Autodesk Fusion 360 part; units mm, degrees
(part 3 of 7)
  line L359 (74.972, -60.812) -> (75.0961, -60.7061)
  line L360 (75.0961, -60.7061) -> (75.2145, -60.5939)
  line L361 (75.2145, -60.5939) -> (75.3268, -60.4755)
  line L362 (75.3268, -60.4755) -> (75.4327, -60.3513)
  line L363 (75.4327, -60.3513) -> (75.6604, -60.5355)
  line L364 (75.6604, -60.5355) -> (75.7298, -60.5765)
  line L365 (75.7298, -60.5765) -> (75.8054, -60.6096)
  line L366 (75.8054, -60.6096) -> (75.8853, -60.6371)
  line L367 (75.8853, -60.6371) -> (75.9686, -60.6597)
  line L368 (75.9686, -60.6597) -> (76.0549, -60.6779)
  line L369 (76.0549, -60.6779) -> (76.1439, -60.6917)
  line L370 (76.1439, -60.6917) -> (76.2354, -60.7014)
  line L371 (76.2354, -60.7014) -> (76.3291, -60.707)
  line L372 (76.3291, -60.707) -> (76.4248, -60.7085)
  line L373 (76.4248, -60.7085) -> (76.5224, -60.7059)
  line L374 (76.5224, -60.7059) -> (76.6217, -60.6994)
  line L375 (76.6217, -60.6994) -> (76.7225, -60.6887)
  line L376 (76.7225, -60.6887) -> (76.7666, -60.6157)
  line L377 (76.7666, -60.6157) -> (76.8092, -60.5419)
  line L378 (76.8092, -60.5419) -> (76.8504, -60.4672)
  line L379 (76.8504, -60.4672) -> (76.8092, -60.3745)
  line L380 (76.8092, -60.3745) -> (76.7652, -60.2853)
  line L381 (76.7652, -60.2853) -> (76.7187, -60.1995)
  line L382 (76.7187, -60.1995) -> (76.6695, -60.1173)
  line L383 (76.6695, -60.1173) -> (76.6178, -60.039)
  line L384 (76.6178, -60.039) -> (76.5637, -59.9646)
  line L385 (76.5637, -59.9646) -> (76.5072, -59.8945)
  line L386 (76.5072, -59.8945) -> (76.4483, -59.8288)
  line L387 (76.4483, -59.8288) -> (76.3871, -59.7679)
  line L388 (76.3871, -59.7679) -> (76.3233, -59.7126)
  line L389 (76.3233, -59.7126) -> (76.2568, -59.6636)
  line L390 (76.2568, -59.6636) -> (76.1866, -59.6241)
  line L391 (76.1866, -59.6241) -> (75.9133, -59.5189)
  line L392 (75.9133, -59.5189) -> (75.9679, -59.3651)
  line L393 (75.9679, -59.3651) -> (76.0142, -59.2086)
  line L394 (76.0142, -59.2086) -> (76.0523, -59.05)
  line L395 (76.0523, -59.05) -> (76.0819, -58.8895)
  circle A0 centre (73.0295, -58.4089) radius 2.2
extrude "Extrude2" add sketch "Sketch2" along normal blind 2 separate body makes body 3 in component "CT idler 1"
combine "Combine1" operation add target body 2 tool bodies 3 makes body 4 at (74.9068, -57.2617, 40.3333) in component "CT idler 1"
ref_plane "WorkPlane1" through (0, 0, 39) normal (0, 0, 1) x (1, 0, 0) in component "CT idler 2"
sketch "Sketch1 (3)" plane through (0, 0, 39) normal (0, 0, 1) x (1, 0, 0) in component "CT idler 2"
  line L0 (68.9168, -62.2983) -> (69.3634, -62.3215)
  line L1 (69.3634, -62.3215) -> (69.4355, -62.319)
  line L2 (69.4355, -62.319) -> (69.5079, -62.3112)
  line L3 (69.5079, -62.3112) -> (69.5805, -62.2999)
  line L4 (69.5805, -62.2999) -> (69.6531, -62.2856)
  line L5 (69.6531, -62.2856) -> (69.7259, -62.2688)
  line L6 (69.7259, -62.2688) -> (69.7986, -62.2497)
  line L7 (69.7986, -62.2497) -> (69.8714, -62.2283)
  line L8 (69.8714, -62.2283) -> (69.9443, -62.205)
  line L9 (69.9443, -62.205) -> (70.0171, -62.1796)
  line L10 (70.0171, -62.1796) -> (70.0898, -62.1524)
  line L11 (70.0898, -62.1524) -> (70.1626, -62.1234)
  line L12 (70.1626, -62.1234) -> (70.2352, -62.0926)
  line L13 (70.2352, -62.0926) -> (70.2374, -61.9521)
  line L14 (70.2374, -61.9521) -> (70.2374, -61.8117)
  line L15 (70.2374, -61.8117) -> (70.2352, -61.6713)
  line L16 (70.2352, -61.6713) -> (70.1626, -61.6405)
  line L17 (70.1626, -61.6405) -> (70.0898, -61.6115)
  line L18 (70.0898, -61.6115) -> (70.0171, -61.5842)
  line L19 (70.0171, -61.5842) -> (69.9443, -61.5589)
  line L20 (69.9443, -61.5589) -> (69.8714, -61.5355)
  line L21 (69.8714, -61.5355) -> (69.7986, -61.5142)
  line L22 (69.7986, -61.5142) -> (69.7259, -61.4951)
  line L23 (69.7259, -61.4951) -> (69.6531, -61.4782)
  line L24 (69.6531, -61.4782) -> (69.5805, -61.464)
  line L25 (69.5805, -61.464) -> (69.5079, -61.4527)
  line L26 (69.5079, -61.4527) -> (69.4355, -61.4449)
  line L27 (69.4355, -61.4449) -> (69.3634, -61.4423)
  line L28 (69.3634, -61.4423) -> (68.9168, -61.4656)
  line L29 (68.9168, -61.4656) -> (68.903, -61.2549)
  line L30 (68.903, -61.2549) -> (68.8837, -61.0447)
  line L31 (68.8837, -61.0447) -> (68.8589, -60.835)
  line L32 (68.8589, -60.835) -> (68.8286, -60.6261)
  line L33 (68.8286, -60.6261) -> (69.2703, -60.5559)
  line L34 (69.2703, -60.5559) -> (69.3403, -60.5385)
  line L35 (69.3403, -60.5385) -> (69.4095, -60.5158)
  line L36 (69.4095, -60.5158) -> (69.4781, -60.4896)
  line L37 (69.4781, -60.4896) -> (69.5462, -60.4606)
  line L38 (69.5462, -60.4606) -> (69.6138, -60.429)
  line L39 (69.6138, -60.429) -> (69.681, -60.3952)
  line L40 (69.681, -60.3952) -> (69.7478, -60.3592)
  line L41 (69.7478, -60.3592) -> (69.8142, -60.3211)
  line L42 (69.8142, -60.3211) -> (69.8801, -60.2812)
  line L43 (69.8801, -60.2812) -> (69.9456, -60.2395)
  line L44 (69.9456, -60.2395) -> (70.0107, -60.1959)
  line L45 (70.0107, -60.1959) -> (70.0754, -60.1507)
  line L46 (70.0754, -60.1507) -> (70.0483, -60.0129)
  line L47 (70.0483, -60.0129) -> (70.0191, -59.8756)
  line L48 (70.0191, -59.8756) -> (69.9878, -59.7387)
  line L49 (69.9878, -59.7387) -> (69.9104, -59.7236)
  line L50 (69.9104, -59.7236) -> (69.8332, -59.7104)
  line L51 (69.8332, -59.7104) -> (69.7563, -59.6989)
  line L52 (69.7563, -59.6989) -> (69.6798, -59.6892)
  line L53 (69.6798, -59.6892) -> (69.6038, -59.6815)
  line L54 (69.6038, -59.6815) -> (69.5281, -59.6758)
  line L55 (69.5281, -59.6758) -> (69.4529, -59.6722)
  line L56 (69.4529, -59.6722) -> (69.3783, -59.6709)
  line L57 (69.3783, -59.6709) -> (69.3043, -59.672)
  line L58 (69.3043, -59.672) -> (69.231, -59.676)
  line L59 (69.231, -59.676) -> (69.1585, -59.6834)
  line L60 (69.1585, -59.6834) -> (69.0875, -59.696)
  line L61 (69.0875, -59.696) -> (68.6554, -59.8116)
  line L62 (68.6554, -59.8116) -> (68.5982, -59.6083)
  line L63 (68.5982, -59.6083) -> (68.5356, -59.4067)
  line L64 (68.5356, -59.4067) -> (68.4677, -59.2068)
  line L65 (68.4677, -59.2068) -> (68.3946, -59.0087)
  line L66 (68.3946, -59.0087) -> (68.812, -58.8483)
  line L67 (68.812, -58.8483) -> (68.8769, -58.8167)
  line L68 (68.8769, -58.8167) -> (68.9399, -58.7801)
  line L69 (68.9399, -58.7801) -> (69.0015, -58.7402)
  line L70 (69.0015, -58.7402) -> (69.0621, -58.6977)
  line L71 (69.0621, -58.6977) -> (69.1217, -58.6527)
  line L72 (69.1217, -58.6527) -> (69.1804, -58.6056)
  line L73 (69.1804, -58.6056) -> (69.2382, -58.5565)
  line L74 (69.2382, -58.5565) -> (69.2952, -58.5056)
  line L75 (69.2952, -58.5056) -> (69.3515, -58.4528)
  line L76 (69.3515, -58.4528) -> (69.4069, -58.3983)
  line L77 (69.4069, -58.3983) -> (69.4615, -58.3422)
  line L78 (69.4615, -58.3422) -> (69.5154, -58.2845)
  line L79 (69.5154, -58.2845) -> (69.4602, -58.1554)
  line L80 (69.4602, -58.1554) -> (69.4031, -58.0271)
  line L81 (69.4031, -58.0271) -> (69.344, -57.8997)
  line L82 (69.344, -57.8997) -> (69.2651, -57.9011)
  line L83 (69.2651, -57.9011) -> (69.1869, -57.9042)
  line L84 (69.1869, -57.9042) -> (69.1093, -57.9089)
  line L85 (69.1093, -57.9089) -> (69.0325, -57.9154)
  line L86 (69.0325, -57.9154) -> (68.9564, -57.9236)
  line L87 (68.9564, -57.9236) -> (68.8813, -57.9338)
  line L88 (68.8813, -57.9338) -> (68.807, -57.9459)
  line L89 (68.807, -57.9459) -> (68.7337, -57.9601)
  line L90 (68.7337, -57.9601) -> (68.6615, -57.9766)
  line L91 (68.6615, -57.9766) -> (68.5907, -57.9958)
  line L92 (68.5907, -57.9958) -> (68.5214, -58.0181)
  line L93 (68.5214, -58.0181) -> (68.4544, -58.0451)
  line L94 (68.4544, -58.0451) -> (68.0559, -58.248)
  line L95 (68.0559, -58.248) -> (67.9576, -58.0611)
  line L96 (67.9576, -58.0611) -> (67.8545, -57.8769)
  line L97 (67.8545, -57.8769) -> (67.7465, -57.6955)
  line L98 (67.7465, -57.6955) -> (67.6338, -57.517)
  line L99 (67.6338, -57.517) -> (68.0088, -57.2733)
  line L100 (68.0088, -57.2733) -> (68.0657, -57.2288)
  line L101 (68.0657, -57.2288) -> (68.1196, -57.1799)
  line L102 (68.1196, -57.1799) -> (68.1717, -57.1281)
  line L103 (68.1717, -57.1281) -> (68.2221, -57.0739)
  line L104 (68.2221, -57.0739) -> (68.271, -57.0176)
  line L105 (68.271, -57.0176) -> (68.3187, -56.9593)
  line L106 (68.3187, -56.9593) -> (68.365, -56.8993)
  line L107 (68.365, -56.8993) -> (68.4102, -56.8375)
  line L108 (68.4102, -56.8375) -> (68.4542, -56.7742)
  line L109 (68.4542, -56.7742) -> (68.4971, -56.7094)
  line L110 (68.4971, -56.7094) -> (68.5389, -56.6432)
  line L111 (68.5389, -56.6432) -> (68.5795, -56.5756)
  line L112 (68.5795, -56.5756) -> (68.4987, -56.4607)
  line L113 (68.4987, -56.4607) -> (68.4162, -56.3471)
  line L114 (68.4162, -56.3471) -> (68.3319, -56.2348)
  line L115 (68.3319, -56.2348) -> (68.255, -56.2526)
  line L116 (68.255, -56.2526) -> (68.1791, -56.2718)
  line L117 (68.1791, -56.2718) -> (68.1043, -56.2926)
  line L118 (68.1043, -56.2926) -> (68.0305, -56.3149)
  line L119 (68.0305, -56.3149) -> (67.9578, -56.3388)
  line L120 (67.9578, -56.3388) -> (67.8864, -56.3643)
  line L121 (67.8864, -56.3643) -> (67.8162, -56.3916)
  line L122 (67.8162, -56.3916) -> (67.7475, -56.4207)
  line L123 (67.7475, -56.4207) -> (67.6804, -56.4519)
  line L124 (67.6804, -56.4519) -> (67.615, -56.4854)
  line L125 (67.615, -56.4854) -> (67.5519, -56.5216)
  line L126 (67.5519, -56.5216) -> (67.492, -56.562)
  line L127 (67.492, -56.562) -> (67.1444, -56.8433)
  line L128 (67.1444, -56.8433) -> (67.0094, -56.6809)
  line L129 (67.0094, -56.6809) -> (66.8702, -56.5222)
  line L130 (66.8702, -56.5222) -> (66.7269, -56.3672)
  line L131 (66.7269, -56.3672) -> (66.5795, -56.216)
  line L132 (66.5795, -56.216) -> (66.8957, -55.8996)
  line L133 (66.8957, -55.8996) -> (66.942, -55.8443)
  line L134 (66.942, -55.8443) -> (66.9847, -55.7853)
  line L135 (66.9847, -55.7853) -> (67.0248, -55.7238)
  line L136 (67.0248, -55.7238) -> (67.0628, -55.6603)
  line L137 (67.0628, -55.6603) -> (67.099, -55.595)
  line L138 (67.099, -55.595) -> (67.1335, -55.5281)
  line L139 (67.1335, -55.5281) -> (67.1663, -55.4597)
  line L140 (67.1663, -55.4597) -> (67.1977, -55.39)
  line L141 (67.1977, -55.39) -> (67.2276, -55.3189)
  line L142 (67.2276, -55.3189) -> (67.256, -55.2466)
  line L143 (67.256, -55.2466) -> (67.2831, -55.1731)
  line L144 (67.2831, -55.1731) -> (67.3089, -55.0985)
  line L145 (67.3089, -55.0985) -> (67.2059, -55.003)
  line L146 (67.2059, -55.003) -> (67.1016, -54.909)
  line L147 (67.1016, -54.909) -> (66.9958, -54.8166)
  line L148 (66.9958, -54.8166) -> (66.9243, -54.85)
  line L149 (66.9243, -54.85) -> (66.854, -54.8847)
  line L150 (66.854, -54.8847) -> (66.7851, -54.9205)
  line L151 (66.7851, -54.9205) -> (66.7176, -54.9577)
  line L152 (66.7176, -54.9577) -> (66.6515, -54.9962)
  line L153 (66.6515, -54.9962) -> (66.5869, -55.036)
  line L154 (66.5869, -55.036) -> (66.524, -55.0773)
  line L155 (66.524, -55.0773) -> (66.4628, -55.1201)
  line L156 (66.4628, -55.1201) -> (66.4036, -55.1645)
  line L157 (66.4036, -55.1645) -> (66.3467, -55.2109)
  line L158 (66.3467, -55.2109) -> (66.2924, -55.2594)
  line L159 (66.2924, -55.2594) -> (66.2423, -55.3113)
  line L160 (66.2423, -55.3113) -> (65.9607, -55.6588)
  line L161 (65.9607, -55.6588) -> (65.7949, -55.528)
  line L162 (65.7949, -55.528) -> (65.6258, -55.4017)
  line L163 (65.6258, -55.4017) -> (65.4534, -55.2799)
  line L164 (65.4534, -55.2799) -> (65.2778, -55.1626)
  line L165 (65.2778, -55.1626) -> (65.5212, -54.7875)
  line L166 (65.5212, -54.7875) -> (65.5551, -54.7237)
  line L167 (65.5551, -54.7237) -> (65.5845, -54.6571)
  line L168 (65.5845, -54.6571) -> (65.611, -54.5886)
  line L169 (65.611, -54.5886) -> (65.635, -54.5186)
  line L170 (65.635, -54.5186) -> (65.6568, -54.4472)
  line L171 (65.6568, -54.4472) -> (65.6766, -54.3746)
  line L172 (65.6766, -54.3746) -> (65.6945, -54.3009)
  line L173 (65.6945, -54.3009) -> (65.7107, -54.2261)
  line L174 (65.7107, -54.2261) -> (65.7251, -54.1504)
  line L175 (65.7251, -54.1504) -> (65.738, -54.0738)
  line L176 (65.738, -54.0738) -> (65.7492, -53.9963)
  line L177 (65.7492, -53.9963) -> (65.7588, -53.9179)
  line L178 (65.7588, -53.9179) -> (65.6383, -53.8459)
  line L179 (65.6383, -53.8459) -> (65.5167, -53.7757)
  line L180 (65.5167, -53.7757) -> (65.394, -53.7073)
  line L181 (65.394, -53.7073) -> (65.331, -53.7549)
  line L182 (65.331, -53.7549) -> (65.2695, -53.8033)
  line L183 (65.2695, -53.8033) -> (65.2095, -53.8527)
  line L184 (65.2095, -53.8527) -> (65.1512, -53.9031)
  line L185 (65.1512, -53.9031) -> (65.0945, -53.9545)
  line L186 (65.0945, -53.9545) -> (65.0397, -54.0069)
  line L187 (65.0397, -54.0069) -> (64.9867, -54.0603)
  line L188 (64.9867, -54.0603) -> (64.9358, -54.1149)
  line L189 (64.9358, -54.1149) -> (64.8871, -54.1707)
  line L190 (64.8871, -54.1707) -> (64.841, -54.2279)
  line L191 (64.841, -54.2279) -> (64.7981, -54.2867)
  line L192 (64.7981, -54.2867) -> (64.7598, -54.3479)
  line L193 (64.7598, -54.3479) -> (64.5566, -54.7463)
  line L194 (64.5566, -54.7463) -> (64.3673, -54.6528)
  line L195 (64.3673, -54.6528) -> (64.1756, -54.5644)
  line L196 (64.1756, -54.5644) -> (63.9816, -54.4811)
  line L197 (63.9816, -54.4811) -> (63.7855, -54.4029)
  line L198 (63.7855, -54.4029) -> (63.9456, -53.9853)
  line L199 (63.9456, -53.9853) -> (63.9655, -53.916)
  line L200 (63.9655, -53.916) -> (63.9804, -53.8447)
  line L201 (63.9804, -53.8447) -> (63.9921, -53.7722)
  line L202 (63.9921, -53.7722) -> (64.001, -53.6987)
  line L203 (64.001, -53.6987) -> (64.0075, -53.6244)
  line L204 (64.0075, -53.6244) -> (64.0117, -53.5492)
  line L205 (64.0117, -53.5492) -> (64.014, -53.4734)
  line L206 (64.014, -53.4734) -> (64.0142, -53.3969)
  line L207 (64.0142, -53.3969) -> (64.0126, -53.3198)
  line L208 (64.0126, -53.3198) -> (64.0092, -53.2422)
  line L209 (64.0092, -53.2422) -> (64.0041, -53.1641)
  line L210 (64.0041, -53.1641) -> (63.9972, -53.0854)
  line L211 (63.9972, -53.0854) -> (63.8644, -53.04)
  line L212 (63.8644, -53.04) -> (63.7308, -52.9966)
  line L213 (63.7308, -52.9966) -> (63.5966, -52.9553)
  line L214 (63.5966, -52.9553) -> (63.5449, -53.0149)
  line L215 (63.5449, -53.0149) -> (63.4948, -53.0751)
  line L216 (63.4948, -53.0751) -> (63.4464, -53.1359)
  line L217 (63.4464, -53.1359) -> (63.3998, -53.1973)
  line L218 (63.3998, -53.1973) -> (63.3551, -53.2593)
  line L219 (63.3551, -53.2593) -> (63.3123, -53.322)
  line L220 (63.3123, -53.322) -> (63.2716, -53.3853)
  line L221 (63.2716, -53.3853) -> (63.2331, -53.4492)
  line L222 (63.2331, -53.4492) -> (63.1971, -53.5139)
  line L223 (63.1971, -53.5139) -> (63.1639, -53.5794)
  line L224 (63.1639, -53.5794) -> (63.1341, -53.6458)
  line L225 (63.1341, -53.6458) -> (63.1094, -53.7137)
  line L226 (63.1094, -53.7137) -> (62.9935, -54.1456)
  line L227 (62.9935, -54.1456) -> (62.7889, -54.0936)
  line L228 (62.7889, -54.0936) -> (62.583, -54.047)
  line L229 (62.583, -54.047) -> (62.3759, -54.0058)
  line L230 (62.3759, -54.0058) -> (62.1678, -53.9701)
  line L231 (62.1678, -53.9701) -> (62.2376, -53.5283)
  line L232 (62.2376, -53.5283) -> (62.2427, -53.4564)
  line L233 (62.2427, -53.4564) -> (62.2425, -53.3835)
  line L234 (62.2425, -53.3835) -> (62.2388, -53.3102)
  line L235 (62.2388, -53.3102) -> (62.2322, -53.2365)
  line L236 (62.2322, -53.2365) -> (62.2231, -53.1624)
  line L237 (62.2231, -53.1624) -> (62.2117, -53.088)
  line L238 (62.2117, -53.088) -> (62.1981, -53.0134)
  line L239 (62.1981, -53.0134) -> (62.1824, -52.9385)
  line L240 (62.1824, -52.9385) -> (62.1648, -52.8635)
  line L241 (62.1648, -52.8635) -> (62.1454, -52.7882)
  line L242 (62.1454, -52.7882) -> (62.1241, -52.7129)
  line L243 (62.1241, -52.7129) -> (62.1011, -52.6374)
  line L244 (62.1011, -52.6374) -> (61.9616, -52.6206)
  line L245 (61.9616, -52.6206) -> (61.822, -52.6059)
  line L246 (61.822, -52.6059) -> (61.6821, -52.5933)
  line L247 (61.6821, -52.5933) -> (61.6439, -52.6624)
  line L248 (61.6439, -52.6624) -> (61.6074, -52.7317)
  line L249 (61.6074, -52.7317) -> (61.5727, -52.8012)
  line L250 (61.5727, -52.8012) -> (61.5399, -52.871)
  line L251 (61.5399, -52.871) -> (61.509, -52.941)
  line L252 (61.509, -52.941) -> (61.4802, -53.0111)
  line L253 (61.4802, -53.0111) -> (61.4536, -53.0815)
  line L254 (61.4536, -53.0815) -> (61.4293, -53.1521)
  line L255 (61.4293, -53.1521) -> (61.4075, -53.2229)
  line L256 (61.4075, -53.2229) -> (61.3886, -53.2938)
  line L257 (61.3886, -53.2938) -> (61.3733, -53.365)
  line L258 (61.3733, -53.365) -> (61.3633, -53.4364)
  line L259 (61.3633, -53.4364) -> (61.3397, -53.8831)
  line L260 (61.3397, -53.8831) -> (61.1287, -53.8747)
  line L261 (61.1287, -53.8747) -> (60.9176, -53.8719)
  line L262 (60.9176, -53.8719) -> (60.7065, -53.8747)
  line L263 (60.7065, -53.8747) -> (60.4956, -53.8831)
  line L264 (60.4956, -53.8831) -> (60.472, -53.4364)
  line L265 (60.472, -53.4364) -> (60.4619, -53.365)
  line L266 (60.4619, -53.365) -> (60.4466, -53.2938)
  line L267 (60.4466, -53.2938) -> (60.4277, -53.2229)
  line L268 (60.4277, -53.2229) -> (60.406, -53.1521)
  line L269 (60.406, -53.1521) -> (60.3817, -53.0815)
  line L270 (60.3817, -53.0815) -> (60.355, -53.0111)
  line L271 (60.355, -53.0111) -> (60.3262, -52.941)
  line L272 (60.3262, -52.941) -> (60.2953, -52.871)
  line L273 (60.2953, -52.871) -> (60.2625, -52.8012)
  line L274 (60.2625, -52.8012) -> (60.2278, -52.7317)
  line L275 (60.2278, -52.7317) -> (60.1914, -52.6624)
  line L276 (60.1914, -52.6624) -> (60.1531, -52.5933)
  line L277 (60.1531, -52.5933) -> (60.0133, -52.6059)
  line L278 (60.0133, -52.6059) -> (59.8736, -52.6206)
  line L279 (59.8736, -52.6206) -> (59.7342, -52.6374)
  line L280 (59.7342, -52.6374) -> (59.7112, -52.7129)
  line L281 (59.7112, -52.7129) -> (59.6899, -52.7882)
  line L282 (59.6899, -52.7882) -> (59.6704, -52.8635)
  line L283 (59.6704, -52.8635) -> (59.6528, -52.9385)
  line L284 (59.6528, -52.9385) -> (59.6372, -53.0134)
  line L285 (59.6372, -53.0134) -> (59.6236, -53.088)
  line L286 (59.6236, -53.088) -> (59.6122, -53.1624)
  line L287 (59.6122, -53.1624) -> (59.603, -53.2365)
  line L288 (59.603, -53.2365) -> (59.5965, -53.3102)
  line L289 (59.5965, -53.3102) -> (59.5928, -53.3835)
  line L290 (59.5928, -53.3835) -> (59.5926, -53.4564)
  line L291 (59.5926, -53.4564) -> (59.5976, -53.5283)
  line L292 (59.5976, -53.5283) -> (59.6674, -53.9701)
  line L293 (59.6674, -53.9701) -> (59.4593, -54.0058)
  line L294 (59.4593, -54.0058) -> (59.2523, -54.047)
  line L295 (59.2523, -54.047) -> (59.0463, -54.0936)
  line L296 (59.0463, -54.0936) -> (58.8417, -54.1456)
  line L297 (58.8417, -54.1456) -> (58.7258, -53.7137)
  line L298 (58.7258, -53.7137) -> (58.7011, -53.6458)
  line L299 (58.7011, -53.6458) -> (58.6713, -53.5794)
  line L300 (58.6713, -53.5794) -> (58.6381, -53.5139)
  line L301 (58.6381, -53.5139) -> (58.6021, -53.4492)
  line L302 (58.6021, -53.4492) -> (58.5637, -53.3853)
  line L303 (58.5637, -53.3853) -> (58.523, -53.322)
  line L304 (58.523, -53.322) -> (58.4802, -53.2593)
  line L305 (58.4802, -53.2593) -> (58.4355, -53.1973)
  line L306 (58.4355, -53.1973) -> (58.3889, -53.1359)
  line L307 (58.3889, -53.1359) -> (58.3405, -53.0751)
  line L308 (58.3405, -53.0751) -> (58.2904, -53.0149)
  line L309 (58.2904, -53.0149) -> (58.2386, -52.9553)
  line L310 (58.2386, -52.9553) -> (58.1044, -52.9966)
  line L311 (58.1044, -52.9966) -> (57.9709, -53.04)
  line L312 (57.9709, -53.04) -> (57.838, -53.0854)
  line L313 (57.838, -53.0854) -> (57.8312, -53.1641)
  line L314 (57.8312, -53.1641) -> (57.826, -53.2422)
  line L315 (57.826, -53.2422) -> (57.8226, -53.3198)
  line L316 (57.8226, -53.3198) -> (57.821, -53.3969)
  line L317 (57.821, -53.3969) -> (57.8213, -53.4734)
  line L318 (57.8213, -53.4734) -> (57.8235, -53.5492)
  line L319 (57.8235, -53.5492) -> (57.8278, -53.6244)
  line L320 (57.8278, -53.6244) -> (57.8343, -53.6987)
  line L321 (57.8343, -53.6987) -> (57.8432, -53.7722)
  line L322 (57.8432, -53.7722) -> (57.8548, -53.8447)
  line L323 (57.8548, -53.8447) -> (57.8698, -53.916)
  line L324 (57.8698, -53.916) -> (57.8896, -53.9853)
  line L325 (57.8896, -53.9853) -> (58.0498, -54.4029)
  line L326 (58.0498, -54.4029) -> (57.8537, -54.4811)
  line L327 (57.8537, -54.4811) -> (57.6597, -54.5644)
  line L328 (57.6597, -54.5644) -> (57.4679, -54.6528)
  line L329 (57.4679, -54.6528) -> (57.2786, -54.7463)
  line L330 (57.2786, -54.7463) -> (57.0754, -54.3479)
  line L331 (57.0754, -54.3479) -> (57.0372, -54.2867)
  line L332 (57.0372, -54.2867) -> (56.9942, -54.2279)
  line L333 (56.9942, -54.2279) -> (56.9481, -54.1707)
  line L334 (56.9481, -54.1707) -> (56.8995, -54.1149)
  line L335 (56.8995, -54.1149) -> (56.8486, -54.0603)
  line L336 (56.8486, -54.0603) -> (56.7956, -54.0069)
  line L337 (56.7956, -54.0069) -> (56.7407, -53.9545)
  line L338 (56.7407, -53.9545) -> (56.6841, -53.9031)
  line L339 (56.6841, -53.9031) -> (56.6257, -53.8527)
  line L340 (56.6257, -53.8527) -> (56.5657, -53.8033)
  line L341 (56.5657, -53.8033) -> (56.5042, -53.7549)
  line L342 (56.5042, -53.7549) -> (56.4412, -53.7073)
  line L343 (56.4412, -53.7073) -> (56.3186, -53.7757)
  line L344 (56.3186, -53.7757) -> (56.1969, -53.8459)
  line L345 (56.1969, -53.8459) -> (56.0764, -53.9179)
  line L346 (56.0764, -53.9179) -> (56.0861, -53.9963)
  line L347 (56.0861, -53.9963) -> (56.0973, -54.0738)
  line L348 (56.0973, -54.0738) -> (56.1101, -54.1504)
  line L349 (56.1101, -54.1504) -> (56.1246, -54.2261)
  line L350 (56.1246, -54.2261) -> (56.1407, -54.3009)
  line L351 (56.1407, -54.3009) -> (56.1587, -54.3746)
  line L352 (56.1587, -54.3746) -> (56.1785, -54.4472)
  line L353 (56.1785, -54.4472) -> (56.2003, -54.5186)
  line L354 (56.2003, -54.5186) -> (56.2243, -54.5886)
  line L355 (56.2243, -54.5886) -> (56.2507, -54.6571)
  line L356 (56.2507, -54.6571) -> (56.2801, -54.7237)
  line L357 (56.2801, -54.7237) -> (56.314, -54.7875)
  line L358 (56.314, -54.7875) -> (56.5575, -55.1626)
  line L359 (56.5575, -55.1626) -> (56.3819, -55.2799)
  line L360 (56.3819, -55.2799) -> (56.2095, -55.4017)
  line L361 (56.2095, -55.4017) -> (56.0403, -55.528)
  line L362 (56.0403, -55.528) -> (55.8745, -55.6588)
  line L363 (55.8745, -55.6588) -> (55.593, -55.3113)
  line L364 (55.593, -55.3113) -> (55.5428, -55.2594)
  line L365 (55.5428, -55.2594) -> (55.4886, -55.2109)
  line L366 (55.4886, -55.2109) -> (55.4316, -55.1645)
  line L367 (55.4316, -55.1645) -> (55.3724, -55.1201)
  line L368 (55.3724, -55.1201) -> (55.3113, -55.0773)
  line L369 (55.3113, -55.0773) -> (55.2483, -55.036)
  line L370 (55.2483, -55.036) -> (55.1838, -54.9962)
  line L371 (55.1838, -54.9962) -> (55.1177, -54.9577)
  line L372 (55.1177, -54.9577) -> (55.0501, -54.9205)
  line L373 (55.0501, -54.9205) -> (54.9812, -54.8847)
  line L374 (54.9812, -54.8847) -> (54.911, -54.85)
  line L375 (54.911, -54.85) -> (54.8394, -54.8166)
  line L376 (54.8394, -54.8166) -> (54.7337, -54.909)
  line L377 (54.7337, -54.909) -> (54.6293, -55.003)
  line L378 (54.6293, -55.003) -> (54.5264, -55.0985)
  line L379 (54.5264, -55.0985) -> (54.5521, -55.1731)
  line L380 (54.5521, -55.1731) -> (54.5792, -55.2466)
  line L381 (54.5792, -55.2466) -> (54.6077, -55.3189)
  line L382 (54.6077, -55.3189) -> (54.6376, -55.39)
  line L383 (54.6376, -55.39) -> (54.6689, -55.4597)
  line L384 (54.6689, -55.4597) -> (54.7018, -55.5281)
  line L385 (54.7018, -55.5281) -> (54.7363, -55.595)
  line L386 (54.7363, -55.595) -> (54.7724, -55.6603)
  line L387 (54.7724, -55.6603) -> (54.8105, -55.7238)
  line L388 (54.8105, -55.7238) -> (54.8506, -55.7853)
  line L389 (54.8506, -55.7853) -> (54.8932, -55.8443)
  line L390 (54.8932, -55.8443) -> (54.9396, -55.8996)
  line L391 (54.9396, -55.8996) -> (55.2557, -56.216)
  line L392 (55.2557, -56.216) -> (55.1084, -56.3672)
  line L393 (55.1084, -56.3672) -> (54.965, -56.5222)
  line L394 (54.965, -56.5222) -> (54.8258, -56.6809)
  line L395 (54.8258, -56.6809) -> (54.6909, -56.8433)
  line L396 (54.6909, -56.8433) -> (54.3432, -56.562)
  line L397 (54.3432, -56.562) -> (54.2834, -56.5216)
  line L398 (54.2834, -56.5216) -> (54.2202, -56.4854)
  line L399 (54.2202, -56.4854) -> (54.1549, -56.4519)
  line L400 (54.1549, -56.4519) -> (54.0877, -56.4207)
  line L401 (54.0877, -56.4207) -> (54.019, -56.3916)
  line L402 (54.019, -56.3916) -> (53.9489, -56.3643)
  line L403 (53.9489, -56.3643) -> (53.8774, -56.3388)
  line L404 (53.8774, -56.3388) -> (53.8048, -56.3149)
  line L405 (53.8048, -56.3149) -> (53.731, -56.2926)
  line L406 (53.731, -56.2926) -> (53.6561, -56.2718)
  line L407 (53.6561, -56.2718) -> (53.5802, -56.2526)
  line L408 (53.5802, -56.2526) -> (53.5033, -56.2348)
  line L409 (53.5033, -56.2348) -> (53.4191, -56.3471)
  line L410 (53.4191, -56.3471) -> (53.3365, -56.4607)
  line L411 (53.3365, -56.4607) -> (53.2557, -56.5756)
  line L412 (53.2557, -56.5756) -> (53.2964, -56.6432)
  line L413 (53.2964, -56.6432) -> (53.3382, -56.7094)
  line L414 (53.3382, -56.7094) -> (53.381, -56.7742)
  line L415 (53.381, -56.7742) -> (53.4251, -56.8375)
  line L416 (53.4251, -56.8375) -> (53.4702, -56.8993)
  line L417 (53.4702, -56.8993) -> (53.5166, -56.9593)
  line L418 (53.5166, -56.9593) -> (53.5642, -57.0176)
  line L419 (53.5642, -57.0176) -> (53.6132, -57.0739)
  line L420 (53.6132, -57.0739) -> (53.6636, -57.1281)
  line L421 (53.6636, -57.1281) -> (53.7156, -57.1799)
  line L422 (53.7156, -57.1799) -> (53.7696, -57.2288)
  line L423 (53.7696, -57.2288) -> (53.8264, -57.2733)
  line L424 (53.8264, -57.2733) -> (54.2014, -57.517)
  line L425 (54.2014, -57.517) -> (54.0887, -57.6955)
  line L426 (54.0887, -57.6955) -> (53.9808, -57.8769)
  line L427 (53.9808, -57.8769) -> (53.8776, -58.0611)
  line L428 (53.8776, -58.0611) -> (53.7794, -58.248)
  line L429 (53.7794, -58.248) -> (53.3808, -58.0451)
  line L430 (53.3808, -58.0451) -> (53.3139, -58.0181)
  line L431 (53.3139, -58.0181) -> (53.2446, -57.9958)
  line L432 (53.2446, -57.9958) -> (53.1737, -57.9766)
  line L433 (53.1737, -57.9766) -> (53.1015, -57.9601)
  line L434 (53.1015, -57.9601) -> (53.0283, -57.9459)
  line L435 (53.0283, -57.9459) -> (52.954, -57.9338)
  line L436 (52.954, -57.9338) -> (52.8788, -57.9236)
  line L437 (52.8788, -57.9236) -> (52.8028, -57.9154)
  line L438 (52.8028, -57.9154) -> (52.7259, -57.9089)
  line L439 (52.7259, -57.9089) -> (52.6484, -57.9042)
  line L440 (52.6484, -57.9042) -> (52.5701, -57.9011)
  line L441 (52.5701, -57.9011) -> (52.4912, -57.8997)
  line L442 (52.4912, -57.8997) -> (52.4322, -58.0271)
  line L443 (52.4322, -58.0271) -> (52.3751, -58.1554)
  line L444 (52.3751, -58.1554) -> (52.3199, -58.2845)
  line L445 (52.3199, -58.2845) -> (52.3737, -58.3422)
  line L446 (52.3737, -58.3422) -> (52.4284, -58.3983)
  line L447 (52.4284, -58.3983) -> (52.4838, -58.4528)
  line L448 (52.4838, -58.4528) -> (52.54, -58.5056)
  line L449 (52.54, -58.5056) -> (52.597, -58.5565)
  line L450 (52.597, -58.5565) -> (52.6549, -58.6056)
  line L451 (52.6549, -58.6056) -> (52.7136, -58.6527)
  line L452 (52.7136, -58.6527) -> (52.7732, -58.6977)
  line L453 (52.7732, -58.6977) -> (52.8337, -58.7402)
  line L454 (52.8337, -58.7402) -> (52.8954, -58.7801)
  line L455 (52.8954, -58.7801) -> (52.9583, -58.8167)
  line L456 (52.9583, -58.8167) -> (53.0232, -58.8483)
  line L457 (53.0232, -58.8483) -> (53.4407, -59.0087)
  line L458 (53.4407, -59.0087) -> (53.3675, -59.2068)
  line L459 (53.3675, -59.2068) -> (53.2997, -59.4067)
  line L460 (53.2997, -59.4067) -> (53.2371, -59.6083)
  line L461 (53.2371, -59.6083) -> (53.1798, -59.8116)
  line L462 (53.1798, -59.8116) -> (52.7478, -59.696)
  line L463 (52.7478, -59.696) -> (52.6767, -59.6834)
  line L464 (52.6767, -59.6834) -> (52.6043, -59.676)
  line L465 (52.6043, -59.676) -> (52.531, -59.672)
  line L466 (52.531, -59.672) -> (52.4569, -59.6709)
  line L467 (52.4569, -59.6709) -> (52.3823, -59.6722)
  line L468 (52.3823, -59.6722) -> (52.3071, -59.6758)
  line L469 (52.3071, -59.6758) -> (52.2315, -59.6815)
  line L470 (52.2315, -59.6815) -> (52.1554, -59.6892)
  line L471 (52.1554, -59.6892) -> (52.0789, -59.6989)
  line L472 (52.0789, -59.6989) -> (52.0021, -59.7104)
  line L473 (52.0021, -59.7104) -> (51.9249, -59.7236)
  line L474 (51.9249, -59.7236) -> (51.8474, -59.7387)
  line L475 (51.8474, -59.7387) -> (51.8161, -59.8756)
  line L476 (51.8161, -59.8756) -> (51.7869, -60.0129)
  line L477 (51.7869, -60.0129) -> (51.7598, -60.1507)
  line L478 (51.7598, -60.1507) -> (51.8245, -60.1959)
  line L479 (51.8245, -60.1959) -> (51.8896, -60.2395)
  line L480 (51.8896, -60.2395) -> (51.9551, -60.2812)
  line L481 (51.9551, -60.2812) -> (52.0211, -60.3211)
  line L482 (52.0211, -60.3211) -> (52.0874, -60.3592)
  line L483 (52.0874, -60.3592) -> (52.1542, -60.3952)
  line L484 (52.1542, -60.3952) -> (52.2214, -60.429)
  line L485 (52.2214, -60.429) -> (52.2891, -60.4606)
  line L486 (52.2891, -60.4606) -> (52.3572, -60.4896)
  line L487 (52.3572, -60.4896) -> (52.4258, -60.5158)
  line L488 (52.4258, -60.5158) -> (52.495, -60.5385)
  line L489 (52.495, -60.5385) -> (52.565, -60.5559)
  line L490 (52.565, -60.5559) -> (53.0067, -60.6261)
  line L491 (53.0067, -60.6261) -> (52.9763, -60.835)
  line L492 (52.9763, -60.835) -> (52.9515, -61.0447)
  line L493 (52.9515, -61.0447) -> (52.9322, -61.2549)
  line L494 (52.9322, -61.2549) -> (52.9185, -61.4656)
  line L495 (52.9185, -61.4656) -> (52.4718, -61.4423)
  line L496 (52.4718, -61.4423) -> (52.3997, -61.4449)
  line L497 (52.3997, -61.4449) -> (52.3273, -61.4527)
  line L498 (52.3273, -61.4527) -> (52.2548, -61.464)
  line L499 (52.2548, -61.464) -> (52.1821, -61.4782)
  line L500 (52.1821, -61.4782) -> (52.1094, -61.4951)
  line L501 (52.1094, -61.4951) -> (52.0366, -61.5142)
  line L502 (52.0366, -61.5142) -> (51.9638, -61.5355)
  line L503 (51.9638, -61.5355) -> (51.891, -61.5589)
  line L504 (51.891, -61.5589) -> (51.8182, -61.5842)
  line L505 (51.8182, -61.5842) -> (51.7454, -61.6115)
  line L506 (51.7454, -61.6115) -> (51.6727, -61.6405)
  line L507 (51.6727, -61.6405) -> (51.6, -61.6713)
  line L508 (51.6, -61.6713) -> (51.5979, -61.8117)
  line L509 (51.5979, -61.8117) -> (51.5979, -61.9521)
  line L510 (51.5979, -61.9521) -> (51.6, -62.0926)
  line L511 (51.6, -62.0926) -> (51.6727, -62.1234)
  line L512 (51.6727, -62.1234) -> (51.7454, -62.1524)
  line L513 (51.7454, -62.1524) -> (51.8182, -62.1796)
  line L514 (51.8182, -62.1796) -> (51.891, -62.205)
  line L515 (51.891, -62.205) -> (51.9638, -62.2283)
  line L516 (51.9638, -62.2283) -> (52.0366, -62.2497)
  line L517 (52.0366, -62.2497) -> (52.1094, -62.2688)
  line L518 (52.1094, -62.2688) -> (52.1821, -62.2856)
  line L519 (52.1821, -62.2856) -> (52.2548, -62.2999)
  line L520 (52.2548, -62.2999) -> (52.3273, -62.3112)
  line L521 (52.3273, -62.3112) -> (52.3997, -62.319)
  line L522 (52.3997, -62.319) -> (52.4718, -62.3215)
  line L523 (52.4718, -62.3215) -> (52.9185, -62.2983)
  line L524 (52.9185, -62.2983) -> (52.9322, -62.509)
  line L525 (52.9322, -62.509) -> (52.9515, -62.7192)
  line L526 (52.9515, -62.7192) -> (52.9763, -62.9289)
  line L527 (52.9763, -62.9289) -> (53.0067, -63.1378)
  line L528 (53.0067, -63.1378) -> (52.565, -63.2079)
  line L529 (52.565, -63.2079) -> (52.495, -63.2254)
  line L530 (52.495, -63.2254) -> (52.4258, -63.2481)
  line L531 (52.4258, -63.2481) -> (52.3572, -63.2742)
  line L532 (52.3572, -63.2742) -> (52.2891, -63.3033)
  line L533 (52.2891, -63.3033) -> (52.2214, -63.3348)
  line L534 (52.2214, -63.3348) -> (52.1542, -63.3687)
  line L535 (52.1542, -63.3687) -> (52.0874, -63.4047)
  line L536 (52.0874, -63.4047) -> (52.0211, -63.4427)
  line L537 (52.0211, -63.4427) -> (51.9551, -63.4826)
  line L538 (51.9551, -63.4826) -> (51.8896, -63.5244)
  line L539 (51.8896, -63.5244) -> (51.8245, -63.5679)
  line L540 (51.8245, -63.5679) -> (51.7598, -63.6131)
  line L541 (51.7598, -63.6131) -> (51.7869, -63.7509)
  line L542 (51.7869, -63.7509) -> (51.8161, -63.8883)
  line L543 (51.8161, -63.8883) -> (51.8474, -64.0252)
  line L544 (51.8474, -64.0252) -> (51.9249, -64.0402)
  line L545 (51.9249, -64.0402) -> (52.0021, -64.0535)
  line L546 (52.0021, -64.0535) -> (52.0789, -64.065)
  line L547 (52.0789, -64.065) -> (52.1554, -64.0746)
  line L548 (52.1554, -64.0746) -> (52.2315, -64.0824)
  line L549 (52.2315, -64.0824) -> (52.3071, -64.0881)
  line L550 (52.3071, -64.0881) -> (52.3823, -64.0917)
  line L551 (52.3823, -64.0917) -> (52.4569, -64.093)
  line L552 (52.4569, -64.093) -> (52.531, -64.0918)
  line L553 (52.531, -64.0918) -> (52.6043, -64.0878)
  line L554 (52.6043, -64.0878) -> (52.6767, -64.0804)
  line L555 (52.6767, -64.0804) -> (52.7478, -64.0679)
  line L556 (52.7478, -64.0679) -> (53.1798, -63.9523)
  line L557 (53.1798, -63.9523) -> (53.2371, -64.1555)
  line L558 (53.2371, -64.1555) -> (53.2997, -64.3572)
  line L559 (53.2997, -64.3572) -> (53.3675, -64.5571)
  line L560 (53.3675, -64.5571) -> (53.4407, -64.7551)
  line L561 (53.4407, -64.7551) -> (53.0232, -64.9156)
  line L562 (53.0232, -64.9156) -> (52.9583, -64.9472)
  line L563 (52.9583, -64.9472) -> (52.8954, -64.9838)
  line L564 (52.8954, -64.9838) -> (52.8337, -65.0236)
  line L565 (52.8337, -65.0236) -> (52.7732, -65.0662)
  line L566 (52.7732, -65.0662) -> (52.7136, -65.1111)
  line L567 (52.7136, -65.1111) -> (52.6549, -65.1582)
  line L568 (52.6549, -65.1582) -> (52.597, -65.2073)
  line L569 (52.597, -65.2073) -> (52.54, -65.2583)
  line L570 (52.54, -65.2583) -> (52.4838, -65.3111)
  line L571 (52.4838, -65.3111) -> (52.4284, -65.3655)
  line L572 (52.4284, -65.3655) -> (52.3737, -65.4216)
  line L573 (52.3737, -65.4216) -> (52.3199, -65.4793)
  line L574 (52.3199, -65.4793) -> (52.3751, -65.6085)
  line L575 (52.3751, -65.6085) -> (52.4322, -65.7368)
  line L576 (52.4322, -65.7368) -> (52.4912, -65.8642)
  line L577 (52.4912, -65.8642) -> (52.5701, -65.8627)
  line L578 (52.5701, -65.8627) -> (52.6484, -65.8597)
  line L579 (52.6484, -65.8597) -> (52.7259, -65.855)
  line L580 (52.7259, -65.855) -> (52.8028, -65.8485)
  line L581 (52.8028, -65.8485) -> (52.8788, -65.8402)
  line L582 (52.8788, -65.8402) -> (52.954, -65.8301)
  line L583 (52.954, -65.8301) -> (53.0283, -65.818)
  line L584 (53.0283, -65.818) -> (53.1015, -65.8038)
  line L585 (53.1015, -65.8038) -> (53.1737, -65.7872)
  line L586 (53.1737, -65.7872) -> (53.2446, -65.7681)
  line L587 (53.2446, -65.7681) -> (53.3139, -65.7458)
  line L588 (53.3139, -65.7458) -> (53.3808, -65.7187)
  line L589 (53.3808, -65.7187) -> (53.7794, -65.5158)
  line L590 (53.7794, -65.5158) -> (53.8776, -65.7027)
  line L591 (53.8776, -65.7027) -> (53.9808, -65.8869)
  line L592 (53.9808, -65.8869) -> (54.0887, -66.0684)
  line L593 (54.0887, -66.0684) -> (54.2014, -66.2469)
  line L594 (54.2014, -66.2469) -> (53.8264, -66.4906)
  line L595 (53.8264, -66.4906) -> (53.7696, -66.535)
  line L596 (53.7696, -66.535) -> (53.7156, -66.5839)
  line L597 (53.7156, -66.5839) -> (53.6636, -66.6357)
  line L598 (53.6636, -66.6357) -> (53.6132, -66.6899)
  line L599 (53.6132, -66.6899) -> (53.5642, -66.7463)
  line L600 (53.5642, -66.7463) -> (53.5166, -66.8046)
  line L601 (53.5166, -66.8046) -> (53.4702, -66.8646)
  line L602 (53.4702, -66.8646) -> (53.4251, -66.9263)
  line L603 (53.4251, -66.9263) -> (53.381, -66.9896)
  line L604 (53.381, -66.9896) -> (53.3382, -67.0544)
  line L605 (53.3382, -67.0544) -> (53.2964, -67.1207)
  line L606 (53.2964, -67.1207) -> (53.2557, -67.1883)
  line L607 (53.2557, -67.1883) -> (53.3365, -67.3031)
  line L608 (53.3365, -67.3031) -> (53.4191, -67.4167)
  line L609 (53.4191, -67.4167) -> (53.5033, -67.5291)
  line L610 (53.5033, -67.5291) -> (53.5802, -67.5113)
  line L611 (53.5802, -67.5113) -> (53.6561, -67.492)
  line L612 (53.6561, -67.492) -> (53.731, -67.4713)
  line L613 (53.731, -67.4713) -> (53.8048, -67.449)
  line L614 (53.8048, -67.449) -> (53.8774, -67.4251)
  line L615 (53.8774, -67.4251) -> (53.9489, -67.3996)
  line L616 (53.9489, -67.3996) -> (54.019, -67.3723)
  line L617 (54.019, -67.3723) -> (54.0877, -67.3431)
  line L618 (54.0877, -67.3431) -> (54.1549, -67.3119)
  line L619 (54.1549, -67.3119) -> (54.2202, -67.2785)
  line L620 (54.2202, -67.2785) -> (54.2834, -67.2422)
  line L621 (54.2834, -67.2422) -> (54.3432, -67.2019)
  line L622 (54.3432, -67.2019) -> (54.6909, -66.9206)
  line L623 (54.6909, -66.9206) -> (54.8258, -67.0829)
  line L624 (54.8258, -67.0829) -> (54.965, -67.2417)
  line L625 (54.965, -67.2417) -> (55.1084, -67.3967)
  line L626 (55.1084, -67.3967) -> (55.2557, -67.5479)
  line L627 (55.2557, -67.5479) -> (54.9396, -67.8642)
  line L628 (54.9396, -67.8642) -> (54.8932, -67.9195)
  line L629 (54.8932, -67.9195) -> (54.8506, -67.9785)
  line L630 (54.8506, -67.9785) -> (54.8105, -68.04)
  line L631 (54.8105, -68.04) -> (54.7724, -68.1036)
  line L632 (54.7724, -68.1036) -> (54.7363, -68.1688)
  line L633 (54.7363, -68.1688) -> (54.7018, -68.2357)
  line L634 (54.7018, -68.2357) -> (54.6689, -68.3041)
  line L635 (54.6689, -68.3041) -> (54.6376, -68.3739)
  line L636 (54.6376, -68.3739) -> (54.6077, -68.4449)
  line L637 (54.6077, -68.4449) -> (54.5792, -68.5172)
  line L638 (54.5792, -68.5172) -> (54.5521, -68.5907)
  line L639 (54.5521, -68.5907) -> (54.5264, -68.6653)
  line L640 (54.5264, -68.6653) -> (54.6293, -68.7609)
  line L641 (54.6293, -68.7609) -> (54.7337, -68.8548)
  line L642 (54.7337, -68.8548) -> (54.8394, -68.9472)
  line L643 (54.8394, -68.9472) -> (54.911, -68.9138)
  line L644 (54.911, -68.9138) -> (54.9812, -68.8792)
  line L645 (54.9812, -68.8792) -> (55.0501, -68.8433)
  line L646 (55.0501, -68.8433) -> (55.1177, -68.8062)
  line L647 (55.1177, -68.8062) -> (55.1838, -68.7677)
  line L648 (55.1838, -68.7677) -> (55.2483, -68.7279)
  line L649 (55.2483, -68.7279) -> (55.3113, -68.6866)
  line L650 (55.3113, -68.6866) -> (55.3724, -68.6438)
  line L651 (55.3724, -68.6438) -> (55.4316, -68.5993)
  line L652 (55.4316, -68.5993) -> (55.4886, -68.553)
  line L653 (55.4886, -68.553) -> (55.5428, -68.5044)
  line L654 (55.5428, -68.5044) -> (55.593, -68.4525)
  line L655 (55.593, -68.4525) -> (55.8745, -68.1051)
  line L656 (55.8745, -68.1051) -> (56.0403, -68.2358)
  line L657 (56.0403, -68.2358) -> (56.2095, -68.3622)
  line L658 (56.2095, -68.3622) -> (56.3819, -68.484)
  line L659 (56.3819, -68.484) -> (56.5575, -68.6012)
  line L660 (56.5575, -68.6012) -> (56.314, -68.9764)
  line L661 (56.314, -68.9764) -> (56.2801, -69.0401)
  line L662 (56.2801, -69.0401) -> (56.2507, -69.1067)
  line L663 (56.2507, -69.1067) -> (56.2243, -69.1752)
  line L664 (56.2243, -69.1752) -> (56.2003, -69.2453)
  line L665 (56.2003, -69.2453) -> (56.1785, -69.3166)
  line L666 (56.1785, -69.3166) -> (56.1587, -69.3892)
  line L667 (56.1587, -69.3892) -> (56.1407, -69.463)
  line L668 (56.1407, -69.463) -> (56.1246, -69.5377)
  line L669 (56.1246, -69.5377) -> (56.1101, -69.6134)
  line L670 (56.1101, -69.6134) -> (56.0973, -69.6901)
  line L671 (56.0973, -69.6901) -> (56.0861, -69.7676)
  line L672 (56.0861, -69.7676) -> (56.0764, -69.8459)
  line L673 (56.0764, -69.8459) -> (56.1969, -69.9179)
  line L674 (56.1969, -69.9179) -> (56.3186, -69.9882)
  line L675 (56.3186, -69.9882) -> (56.4412, -70.0565)
  line L676 (56.4412, -70.0565) -> (56.5042, -70.009)
  line L677 (56.5042, -70.009) -> (56.5657, -69.9605)
  line L678 (56.5657, -69.9605) -> (56.6257, -69.9111)
  line L679 (56.6257, -69.9111) -> (56.6841, -69.8607)
  line L680 (56.6841, -69.8607) -> (56.7407, -69.8094)
  line L681 (56.7407, -69.8094) -> (56.7956, -69.757)
  line L682 (56.7956, -69.757) -> (56.8486, -69.7035)
  line L683 (56.8486, -69.7035) -> (56.8995, -69.6489)
  line L684 (56.8995, -69.6489) -> (56.9481, -69.5931)
  line L685 (56.9481, -69.5931) -> (56.9942, -69.536)
  line L686 (56.9942, -69.536) -> (57.0372, -69.4772)
  line L687 (57.0372, -69.4772) -> (57.0754, -69.416)
  line L688 (57.0754, -69.416) -> (57.2786, -69.0176)
  line L689 (57.2786, -69.0176) -> (57.4679, -69.111)
  line L690 (57.4679, -69.111) -> (57.6597, -69.1994)
  line L691 (57.6597, -69.1994) -> (57.8537, -69.2828)
  line L692 (57.8537, -69.2828) -> (58.0498, -69.3609)
  line L693 (58.0498, -69.3609) -> (57.8896, -69.7785)
  line L694 (57.8896, -69.7785) -> (57.8698, -69.8479)
  line L695 (57.8698, -69.8479) -> (57.8548, -69.9192)
  line L696 (57.8548, -69.9192) -> (57.8432, -69.9916)
  line L697 (57.8432, -69.9916) -> (57.8343, -70.0651)
  line L698 (57.8343, -70.0651) -> (57.8278, -70.1395)
  line L699 (57.8278, -70.1395) -> (57.8235, -70.2146)
  line L700 (57.8235, -70.2146) -> (57.8213, -70.2905)
  line L701 (57.8213, -70.2905) -> (57.821, -70.3669)
  line L702 (57.821, -70.3669) -> (57.8226, -70.444)
  line L703 (57.8226, -70.444) -> (57.826, -70.5217)
  line L704 (57.826, -70.5217) -> (57.8312, -70.5998)
  line L705 (57.8312, -70.5998) -> (57.838, -70.6784)
  line L706 (57.838, -70.6784) -> (57.9709, -70.7238)
  line L707 (57.9709, -70.7238) -> (58.1044, -70.7672)
  line L708 (58.1044, -70.7672) -> (58.2386, -70.8086)
  line L709 (58.2386, -70.8086) -> (58.2904, -70.749)
  line L710 (58.2904, -70.749) -> (58.3405, -70.6888)
  line L711 (58.3405, -70.6888) -> (58.3889, -70.628)
  line L712 (58.3889, -70.628) -> (58.4355, -70.5666)
  line L713 (58.4355, -70.5666) -> (58.4802, -70.5046)
  line L714 (58.4802, -70.5046) -> (58.523, -70.4419)
  line L715 (58.523, -70.4419) -> (58.5637, -70.3786)
  line L716 (58.5637, -70.3786) -> (58.6021, -70.3146)
  line L717 (58.6021, -70.3146) -> (58.6381, -70.2499)
  line L718 (58.6381, -70.2499) -> (58.6713, -70.1844)
  line L719 (58.6713, -70.1844) -> (58.7011, -70.118)
  line L720 (58.7011, -70.118) -> (58.7258, -70.0502)
  line L721 (58.7258, -70.0502) -> (58.8417, -69.6183)
  line L722 (58.8417, -69.6183) -> (59.0463, -69.6703)
  line L723 (59.0463, -69.6703) -> (59.2523, -69.7169)
  line L724 (59.2523, -69.7169) -> (59.4593, -69.7581)
  line L725 (59.4593, -69.7581) -> (59.6674, -69.7938)
  line L726 (59.6674, -69.7938) -> (59.5976, -70.2355)
  line L727 (59.5976, -70.2355) -> (59.5926, -70.3075)
  line L728 (59.5926, -70.3075) -> (59.5928, -70.3803)
  line L729 (59.5928, -70.3803) -> (59.5965, -70.4536)
  line L730 (59.5965, -70.4536) -> (59.603, -70.5274)
  line L731 (59.603, -70.5274) -> (59.6122, -70.6015)
  line L732 (59.6122, -70.6015) -> (59.6236, -70.6758)
  line L733 (59.6236, -70.6758) -> (59.6372, -70.7505)
  line L734 (59.6372, -70.7505) -> (59.6528, -70.8253)
  line L735 (59.6528, -70.8253) -> (59.6704, -70.9004)
  line L736 (59.6704, -70.9004) -> (59.6899, -70.9756)
  line L737 (59.6899, -70.9756) -> (59.7112, -71.051)
  line L738 (59.7112, -71.051) -> (59.7342, -71.1265)
  line L739 (59.7342, -71.1265) -> (59.8736, -71.1433)
  line L740 (59.8736, -71.1433) -> (60.0133, -71.158)
  line L741 (60.0133, -71.158) -> (60.1531, -71.1705)
  line L742 (60.1531, -71.1705) -> (60.1914, -71.1015)
  line L743 (60.1914, -71.1015) -> (60.2278, -71.0322)
  line L744 (60.2278, -71.0322) -> (60.2625, -70.9626)
  line L745 (60.2625, -70.9626) -> (60.2953, -70.8929)
  line L746 (60.2953, -70.8929) -> (60.3262, -70.8229)
  line L747 (60.3262, -70.8229) -> (60.355, -70.7527)
  line L748 (60.355, -70.7527) -> (60.3817, -70.6823)
  line L749 (60.3817, -70.6823) -> (60.406, -70.6118)
  line L750 (60.406, -70.6118) -> (60.4277, -70.541)
  line L751 (60.4277, -70.541) -> (60.4466, -70.4701)
  line L752 (60.4466, -70.4701) -> (60.4619, -70.3989)
  line L753 (60.4619, -70.3989) -> (60.472, -70.3274)
  line L754 (60.472, -70.3274) -> (60.4956, -69.8808)
  line L755 (60.4956, -69.8808) -> (60.7065, -69.8891)
  line L756 (60.7065, -69.8891) -> (60.9176, -69.8919)
  line L757 (60.9176, -69.8919) -> (61.1287, -69.8891)
  line L758 (61.1287, -69.8891) -> (61.3397, -69.8808)
  line L759 (61.3397, -69.8808) -> (61.3633, -70.3274)
  line L760 (61.3633, -70.3274) -> (61.3733, -70.3989)
  line L761 (61.3733, -70.3989) -> (61.3886, -70.4701)
  line L762 (61.3886, -70.4701) -> (61.4075, -70.541)
  line L763 (61.4075, -70.541) -> (61.4293, -70.6118)
  line L764 (61.4293, -70.6118) -> (61.4536, -70.6823)
  line L765 (61.4536, -70.6823) -> (61.4802, -70.7527)
  line L766 (61.4802, -70.7527) -> (61.509, -70.8229)
  line L767 (61.509, -70.8229) -> (61.5399, -70.8929)
  line L768 (61.5399, -70.8929) -> (61.5727, -70.9626)
  line L769 (61.5727, -70.9626) -> (61.6074, -71.0322)
  line L770 (61.6074, -71.0322) -> (61.6439, -71.1015)
  line L771 (61.6439, -71.1015) -> (61.6821, -71.1705)
  line L772 (61.6821, -71.1705) -> (61.822, -71.158)
  line L773 (61.822, -71.158) -> (61.9616, -71.1433)
  line L774 (61.9616, -71.1433) -> (62.1011, -71.1265)
  line L775 (62.1011, -71.1265) -> (62.1241, -71.051)
  line L776 (62.1241, -71.051) -> (62.1454, -70.9756)
  line L777 (62.1454, -70.9756) -> (62.1648, -70.9004)
  line L778 (62.1648, -70.9004) -> (62.1824, -70.8253)
  line L779 (62.1824, -70.8253) -> (62.1981, -70.7505)
  line L780 (62.1981, -70.7505) -> (62.2117, -70.6758)
  line L781 (62.2117, -70.6758) -> (62.2231, -70.6015)
  line L782 (62.2231, -70.6015) -> (62.2322, -70.5274)
  line L783 (62.2322, -70.5274) -> (62.2388, -70.4536)
  line L784 (62.2388, -70.4536) -> (62.2425, -70.3803)
  line L785 (62.2425, -70.3803) -> (62.2427, -70.3075)
  line L786 (62.2427, -70.3075) -> (62.2376, -70.2355)
  line L787 (62.2376, -70.2355) -> (62.1678, -69.7938)
  line L788 (62.1678, -69.7938) -> (62.3759, -69.7581)
  line L789 (62.3759, -69.7581) -> (62.583, -69.7169)
  line L790 (62.583, -69.7169) -> (62.7889, -69.6703)
  line L791 (62.7889, -69.6703) -> (62.9935, -69.6183)
  line L792 (62.9935, -69.6183) -> (63.1094, -70.0502)
  line L793 (63.1094, -70.0502) -> (63.1341, -70.118)
  line L794 (63.1341, -70.118) -> (63.1639, -70.1844)
  line L795 (63.1639, -70.1844) -> (63.1971, -70.2499)
  line L796 (63.1971, -70.2499) -> (63.2331, -70.3146)
  line L797 (63.2331, -70.3146) -> (63.2716, -70.3786)
  line L798 (63.2716, -70.3786) -> (63.3123, -70.4419)
  line L799 (63.3123, -70.4419) -> (63.3551, -70.5046)
  line L800 (63.3551, -70.5046) -> (63.3998, -70.5666)
  line L801 (63.3998, -70.5666) -> (63.4464, -70.628)
  line L802 (63.4464, -70.628) -> (63.4948, -70.6888)
  line L803 (63.4948, -70.6888) -> (63.5449, -70.749)
  line L804 (63.5449, -70.749) -> (63.5966, -70.8086)
  line L805 (63.5966, -70.8086) -> (63.7308, -70.7672)
  line L806 (63.7308, -70.7672) -> (63.8644, -70.7238)
  line L807 (63.8644, -70.7238) -> (63.9972, -70.6784)
  line L808 (63.9972, -70.6784) -> (64.0041, -70.5998)
  line L809 (64.0041, -70.5998) -> (64.0092, -70.5217)
  line L810 (64.0092, -70.5217) -> (64.0126, -70.444)
  line L811 (64.0126, -70.444) -> (64.0142, -70.3669)
  line L812 (64.0142, -70.3669) -> (64.014, -70.2905)
  line L813 (64.014, -70.2905) -> (64.0117, -70.2146)
  line L814 (64.0117, -70.2146) -> (64.0075, -70.1395)
  line L815 (64.0075, -70.1395) -> (64.001, -70.0651)
  line L816 (64.001, -70.0651) -> (63.9921, -69.9916)
  line L817 (63.9921, -69.9916) -> (63.9804, -69.9192)
  line L818 (63.9804, -69.9192) -> (63.9655, -69.8479)
  line L819 (63.9655, -69.8479) -> (63.9456, -69.7785)
  line L820 (63.9456, -69.7785) -> (63.7855, -69.3609)
  line L821 (63.7855, -69.3609) -> (63.9816, -69.2828)
  line L822 (63.9816, -69.2828) -> (64.1756, -69.1994)
  line L823 (64.1756, -69.1994) -> (64.3673, -69.111)
  line L824 (64.3673, -69.111) -> (64.5566, -69.0176)
  line L825 (64.5566, -69.0176) -> (64.7598, -69.416)
  line L826 (64.7598, -69.416) -> (64.7981, -69.4772)
  line L827 (64.7981, -69.4772) -> (64.841, -69.536)
  line L828 (64.841, -69.536) -> (64.8871, -69.5931)
  line L829 (64.8871, -69.5931) -> (64.9358, -69.6489)
  line L830 (64.9358, -69.6489) -> (64.9867, -69.7035)
  line L831 (64.9867, -69.7035) -> (65.0397, -69.757)
  line L832 (65.0397, -69.757) -> (65.0945, -69.8094)
  line L833 (65.0945, -69.8094) -> (65.1512, -69.8607)
  line L834 (65.1512, -69.8607) -> (65.2095, -69.9111)
  line L835 (65.2095, -69.9111) -> (65.2695, -69.9605)
  line L836 (65.2695, -69.9605) -> (65.331, -70.009)
  line L837 (65.331, -70.009) -> (65.394, -70.0565)
  line L838 (65.394, -70.0565) -> (65.5167, -69.9882)
  line L839 (65.5167, -69.9882) -> (65.6383, -69.9179)
  line L840 (65.6383, -69.9179) -> (65.7588, -69.8459)
  line L841 (65.7588, -69.8459) -> (65.7492, -69.7676)
  line L842 (65.7492, -69.7676) -> (65.738, -69.6901)
  line L843 (65.738, -69.6901) -> (65.7251, -69.6134)
  line L844 (65.7251, -69.6134) -> (65.7107, -69.5377)
  line L845 (65.7107, -69.5377) -> (65.6945, -69.463)
  line L846 (65.6945, -69.463) -> (65.6766, -69.3892)
  line L847 (65.6766, -69.3892) -> (65.6568, -69.3166)
  line L848 (65.6568, -69.3166) -> (65.635, -69.2453)
  line L849 (65.635, -69.2453) -> (65.611, -69.1752)
  line L850 (65.611, -69.1752) -> (65.5845, -69.1067)
  line L851 (65.5845, -69.1067) -> (65.5551, -69.0401)
  line L852 (65.5551, -69.0401) -> (65.5212, -68.9764)
  line L853 (65.5212, -68.9764) -> (65.2778, -68.6012)
  line L854 (65.2778, -68.6012) -> (65.4534, -68.484)
  line L855 (65.4534, -68.484) -> (65.6258, -68.3622)
  line L856 (65.6258, -68.3622) -> (65.7949, -68.2358)
  line L857 (65.7949, -68.2358) -> (65.9607, -68.1051)
  line L858 (65.9607, -68.1051) -> (66.2423, -68.4525)
  line L859 (66.2423, -68.4525) -> (66.2924, -68.5044)
  line L860 (66.2924, -68.5044) -> (66.3467, -68.553)
  line L861 (66.3467, -68.553) -> (66.4036, -68.5993)
  line L862 (66.4036, -68.5993) -> (66.4628, -68.6438)
  line L863 (66.4628, -68.6438) -> (66.524, -68.6866)
  line L864 (66.524, -68.6866) -> (66.5869, -68.7279)
  line L865 (66.5869, -68.7279) -> (66.6515, -68.7677)
  line L866 (66.6515, -68.7677) -> (66.7176, -68.8062)
  line L867 (66.7176, -68.8062) -> (66.7851, -68.8433)
  line L868 (66.7851, -68.8433) -> (66.854, -68.8792)
  line L869 (66.854, -68.8792) -> (66.9243, -68.9138)